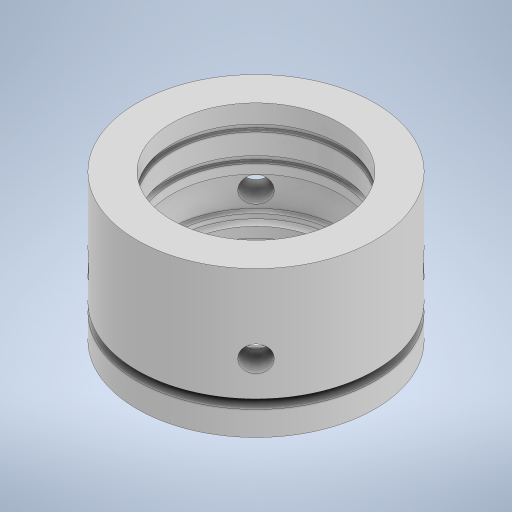
# Autodesk Inventor part: 1 Wash Chamber Conduit
Saved by Autodesk Inventor 2024 (Build 280153000, 153)
## iProperties
Created: 2024-04-17
Part Number: 1 Wash Chamber Conduit
Material: Generic
Document SubType Name: Modeling
Designer: Tommy Rohmann
Density: 1 g/cm^3
Appearance: Default
Author: Tommy Rohmann
Autodesk Inventor part; units mm, degrees
ref_plane "YZ Plane" through (0, 0, 0) normal (1, 0, 0) x (0, 1, 0)
ref_plane "XZ Plane" through (0, 0, 0) normal (0, 1, 0) x (-1, 0, 0)
ref_plane "XY Plane" through (0, 0, 0) normal (0, 0, 1) x (1, 0, 0)
sketch "Sketch1" plane through (0, 0, 0) normal (0, 0, 1) x (1, 0, 0)
  line L0 (0, 0) -> (0, 264.7381)
  line L1 (0, 0) -> (226.2902, 0)
  line L2 (57.15, 111.6982) -> (57.15, -43.1569) construction
  line L3 (57.15, 88.9) -> (61.9125, 88.9)
  line L4 (61.9125, 88.9) -> (61.9125, 84.1375)
  line L5 (61.9125, 84.1375) -> (57.15, 84.1375)
  line L6 (58.42, 111.6982) -> (58.42, -43.1569)
  line L7 (57.15, 69.8915) -> (61.9125, 69.8915)
  line L8 (61.9125, 69.8915) -> (61.9125, 65.129)
  line L9 (61.9125, 65.129) -> (57.15, 65.129)
  line L10 (82.55, -31.5879) -> (82.55, 132.369)
  line L11 (57.15, 58.779) -> (82.55, 58.779)
  line L12 (-11.0868, 101.6) -> (137.3621, 101.6)
  line L13 (67.31, 48.619) -> (57.15, 48.619) construction
  line L14 (82.55, 35.919) -> (57.15, 35.919)
  line L15 (67.31, 35.919) -> (67.31, 101.6)
  line L16 (0, 23.219) -> (113.1451, 23.219)
  line L17 (50.8, -9.4325) -> (50.8, 125.2146)
  line L18 (55.1814, 16.869) -> (109.5306, 16.869)
  line L19 (69.85, 45.922) -> (69.85, 0)
  line L20 (39.3044, 32.744) -> (103.4238, 32.744)
  line L21 (53.5107, 8.89) -> (72.7159, 8.89)
  line L22 (61.9252, 8.89) -> (61.9252, 13.6652)
  line L23 (61.9252, 13.6652) -> (57.15, 13.6652)
  line L24 (50.8, 32.744) -> (62.3413, 0)
  line L25 (53.975, -5.93) -> (53.975, 45.922)
  line L26 (50.323, 18.4438) -> (69.5282, 18.4438)
  line L27 (58.7375, 18.4438) -> (58.7375, 23.219)
  line L28 (58.7375, 23.219) -> (53.9623, 23.219)
  line L29 (61.595, 29.7896) -> (61.595, 62.5774)
  line L30 (57.15, 35.919) -> (57.15, 32.744)
  point P0 (58.42, 84.1375)
  point P1 (58.42, 69.8915)
  point P2 (58.42, 65.129)
  point P3 (82.55, 0)
  point P4 (82.55, 101.6)
  point P5 (58.42, 101.6)
  point P6 (58.42, 88.9)
  point P7 (0, 101.6)
  point P8 (58.42, 0)
  point P9 (58.42, 58.779)
  point P10 (67.31, 58.779)
  point P11 (67.31, 39.0923)
  point P12 (50.8, 23.219)
  point P13 (50.8, 0)
  point P14 (50.8, 101.6)
  point P15 (58.42, 23.219)
  point P16 (82.55, 23.219)
  point P17 (82.55, 16.869)
  point P18 (69.85, 16.869)
  point P19 (69.85, 23.219)
  point P20 (58.42, 35.919)
  point P21 (58.42, 16.869)
  point P22 (69.85, 35.919)
  point P23 (58.42, 32.744)
  point P24 (50.8, 39.0923)
  point P25 (69.85, 32.744)
  point P26 (82.55, 32.744)
  point P27 (57.5247, 13.6652)
  point P28 (59.2078, 8.89)
  point P29 (54.1573, 23.219)
  point P30 (58.42, 18.4438)
  point P31 (55.8404, 18.4438)
  point P32 (61.595, 58.779)
  point P33 (61.595, 35.919)
  dimension "d5" = 57.15
  dimension "d6" = 4.7625
  dimension "d7" = 4.7625
  dimension "d8" = 1.27
  dimension "d10" = 4.7625
  dimension "d11" = 4.7625
  dimension "d12" = 14.246
  dimension "d13" = 82.55
  dimension "d14" = 12.7
  dimension "d15" = 6.35
  dimension "d16" = 10.16
  dimension "d17" = 12.7
  dimension "d18" = 15.24
  dimension "d20" = 12.7
  dimension "d21" = 50.8
  dimension "d22" = 6.35
  dimension "d23" = 12.7
  dimension "d31" = 3.175
  dimension "d40" = 8.89
  dimension "d41" = 101.6
  dimension "d42" = 4.7752
  dimension "d43" = 4.7752
  dimension "d44" = 53.975
  dimension "d45" = 4.7752
  dimension "d46" = 58.7375
  dimension "d50" = 3.175
  constraints: 60 end point, 13 point on line, 12 horizontal, 11 vertical, 4 perpendicular, 10 other
  measures "d6" distance of L3.end L4.end
  measures "d7" distance of L3.start L3.end
  measures "d10" distance of L7.end L8.end
  measures "d11" distance of L7.start L7.end
  measures "d12" distance between parallel lines of L5 L7
  measures "d13" distance between parallel lines of L0 L10
  measures "d14" distance between parallel lines of L3 L12
  measures "d15" distance between parallel lines of L9 L11
  measures "d16" distance between parallel lines of L13 L11
  measures "d17" distance between parallel lines of L13 L14
  measures "d18" distance between parallel lines of L10 L15
  measures "d20" distance between parallel lines of L14 L16
  measures "d21" distance between parallel lines of L0 L17
  measures "d22" distance between parallel lines of L18 L16
  measures "d23" distance between parallel lines of L10 L19
  measures "d31" distance between parallel lines of L14 L20
  measures "d40" distance between parallel lines of L1 L21
  measures "d41" distance between parallel lines of L1 L12
  measures "d42" distance of L22.start L22.end
  measures "d43" length of L22
  measures "d44" distance between parallel lines of L0 L25
  measures "d45" distance of L27.start L28.start
  measures "d46" distance between parallel lines of L0 L27
  measures "d50" distance between parallel lines of L6 L29
revolve "Revolution1" add sketch "Sketch1" angle 90 about axis through (0, 0, 0) along (0, 1, 0) contours L20 L25 L24 | L12 L15 L11 L6 L9 L8 L7 L5 L4 L3 | L20 L6 L16 L24 L25 | L24 L21 L19 L1 | L26 L6 L18 L24 | L12 L10 L11 L15 | L30 L14 L6 L20 | L19 L18 L10 L1 | L18 L6 L23 L24 | L26 L27 L16 L19 L18 L6 | L6 L16 L27 L26 | L15 L14 L29 L11 | L11 L10 L14 L15 | L6 L20 L19 L16 | L6 L14 L29 L20 | L21 L22 L23 L6 L18 L19 | L14 L19 L20 L29 | L10 L20 L19 L14 | L19 L20 L10 L16
ref_plane "Work Plane2" through (61.595, 62.5774, 0) normal (0.7071068, 0, -0.7071068) x (0, -1, 0)
sketch "Sketch5" plane through (61.595, 62.5774, 0) normal (0.7071068, 0, -0.7071068) x (0, -1, 0)
  line L0 (3.7984, 0) -> (26.6584, 0) projected
  line L1 (15.2284, 0) -> (15.2284, 87.1085)
  line L2 (26.6584, 87.1085) -> (3.7984, 87.1085) projected
  circle A0 centre (15.2284, 43.5542) radius 8.9297
  point P0 (62.5774, 43.5542)
  dimension "d52" = 17.8594
  constraints: 3 midpoint, 2 end point, 1 centre point
  measures "d52" diameter of A0
extrude "Extrusion3" cut sketch "Sketch5" along normal blind 160.3375
pattern_circular "Circular Pattern3" count 4 over 360 about axis through (0, -10, 0) along (0, 1, 0)
equation "\"d7\" = d6"
equation "\"d11\" = d10"
equation "\"d43\" = d42"
body "Solid1"
